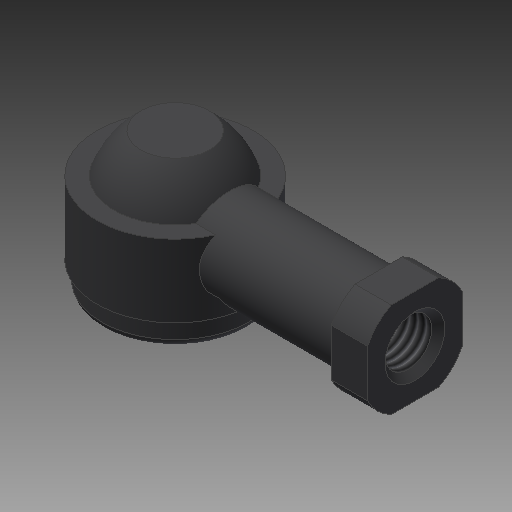
# Autodesk Inventor part: LHSA 10 Body1
Saved by Autodesk Inventor 2018 (Build 220112000, 112)
## iProperties
Category: PARTsolutions
Company: IKO
Created: 2017-10-01
Part Number: LHSA 10 Body1
Catalog Web Link: www.cadenas.de
Description: LHSA B1-
Vendor: IKO
Document SubType Name: Modeling
Designer: psAdmin
Manufacturer: IKO
Mass: 10.6246 g
Surface Area: 72.686 cm^2
Volume: 10.6246 cm^3
Density: 1 g/cm^3
Material: 一般
Appearance: PSOLRGB-128-128-128
PSOL_IDENT_0: {$CADENAS_DATA\23d-libs\iko\iko_bearings\l_balls\lhsa_body.prj},169 {VTYP=3D},{NB=LHSA 10 Body1},{LI
PSOL_IDENT_1: NA=LHSA 10 Body1},{NN=LHSA B1},{DATE=13.10.2016 10:02:12},{GEOMDATE=06.12.2007 08:55:00},{VERSION=},
PSOL_IDENT_2: {LINEID=60},{LINESUBID=-1},{WBVAR=}  {NB=LHSA 10 Body1},{LINA=LHSA 10 Body1},{KT=DUMMY},{IDNR=},{ORD
PSOL_IDENT_3: ER=LHSA 10},{VERS=3},{RID=G_50},{STDRT=10},{DESCR=LHSA},{TRNUMBER=},{PAST=A},{REST=O},{MASS=106},{S=
PSOL_IDENT_4: M10x1.25},{KDM=8.647},{NDM=10.000},{P1=1.250},{V=10},{D=28},{L=57.0},{L1=43},{L2=23},{SL1=6.5},{W=17
PSOL_IDENT_5: },{W1=17},{W2=17},{D1=15.0},{D2=19},{LL=49.0},{P=12.0},{LL1=16.0},{LL2=21.0},{LL3=17.0},{SDK=19.050}
PSOL_IDENT_6: ,{V1=11.0},{D3=12.2475},{D4=21.2001},{D5=26.3},{D6=25.65},{L3=53.8825},{L4=26.1906},{L5=28.5},{L12=3
PSOL_IDENT_7: 0.1645},{B=8.5},{B1=5.0},{B2=6.5},{B3=11.5},{B4=13.0},{B5=17.5073},{LL4=4.5},{LL5=9.0},{CB=0.0},{CC=
PSOL_IDENT_8: 0.9},{E=0},{F=0.0},{C1=1.1765},{C2=1.0},{R1=5},{R2=34.5114},{R3=15.7},{R4=1.3},{CS=7400},{SS1=8.160}
PSOL_IDENT_9: ,{S1=10},{LX=25},{LX1=28.0},{BL=3},{SC=1}
NN: LHSA B1
NB: LHSA 10 Body1
NBSYN: $ORDER. Body1
LINA: LHSA 10 Body1
ORDER: LHSA 10
VERS: 3
RID: G_50
STDRT: 10
DESCR: LHSA
PAST: A
REST: O
MASS: 106
S: M10x1.25
NDM: 10.000
P1: 1.250
V: 10
D: 28
L: 57.0
L1: 43
L2: 23
SL1: 6.5
W: 17
W1: 17
W2: 17
D1: 15.0
D2: 19
LL: 49.0
P: 12.0
LL1: 16.0
LL2: 21.0
LL3: 17.0
SDK: 19.050
V1: 11.0
D3: 12.2475
D4: 21.2001
D5: 26.3
D6: 25.65
L3: 53.8825
L4: 26.1906
L5: 28.5
L12: 30.1645
B: 8.5
B1: 5.0
B2: 6.5
B3: 11.5
B4: 13.0
B5: 17.5073
LL4: 4.5
LL5: 9.0
CB: 0.0
CC: 0.9
E: 0
F: 0.0
C1: 1.1765
C2: 1.0
R1: 5
R2: 34.5114
R3: 15.7
R4: 1.3
CS: 7400
SS1: 8.160
S1: 10
LX: 25
LX1: 28.0
BL: 3
SC: 1
SUPPLIER: IKO
ARTICLENO: LHSA 10 Body1
BOMINFO: LHSA 10 Body1
CREATOR: CADENAS GmbH
Title: LHSA 10 Body1
Author: Cadenas PARTsolutions
Autodesk Inventor part; units mm, degrees
sketch "Sketch_2" plane through (0, 0, 0) normal (0, 0, 1) x (1, 0, 0)
  line L0 (43, 16) -> (0, 16)
  line L1 (0, 16) -> (0, 23.5)
  line L2 (0, 23.5) -> (36.5, 23.5)
  line L3 (36.5, 23.5) -> (36.5, 25.5)
  line L4 (36.5, 25.5) -> (43, 25.5)
  line L5 (43, 25.5) -> (43, 16)
  line L6 (43, 16) -> (0, 16)
  constraints: 14 end point
revolve "Revolution1" add sketch "Sketch_2" angle 360 about axis through (43, 16, 0) along (1, 0, 0)
sketch "Sketch_16" plane through (0, 0, 0) normal (0, 0, 1) x (1, 0, 0)
  line L0 (-14, 12.5) -> (-14, 4.7)
  line L1 (-14, 4.7) -> (45.85, 4.7)
  line L2 (45.85, 4.7) -> (45.85, 27.3)
  line L3 (45.85, 27.3) -> (16.8094, 27.3)
  line L4 (16.8094, 27.3) -> (16.8094, 23.5)
  line L5 (16.8094, 23.5) -> (36.5, 23.5)
  line L6 (36.5, 23.5) -> (36.5, 24.5)
  line L7 (36.5, 24.5) -> (43, 24.5)
  line L8 (43, 24.5) -> (43, 7.5)
  line L9 (43, 7.5) -> (36.5, 7.5)
  line L10 (36.5, 7.5) -> (36.5, 8.5)
  line L11 (36.5, 8.5) -> (16.8094, 8.5)
  line L12 (16.8094, 8.5) -> (14.5, 12.5)
  line L13 (14.5, 12.5) -> (-14, 12.5)
  constraints: 28 end point
extrude "Extrusion1" cut sketch "Sketch_16" along normal mid plane 38
sketch "Sketch_12" plane through (0, 0, 0) normal (0, 0, 1) x (1, 0, 0)
  line L0 (0, 9.5) -> (0, 28)
  line L1 (0, 28) -> (6.1238, 28)
  arc A0 (10.8825, 21) -> (6.1238, 28) centre (-4.0001, 16.0001) ccw
  line L2 (10.8825, 21) -> (14, 21)
  line L3 (14, 21) -> (14, 12.5)
  line L4 (14, 12.5) -> (12.825, 12.5)
  line L5 (12.825, 12.5) -> (12.825, 9.5)
  line L6 (12.825, 9.5) -> (0, 9.5)
  line L7 (0, 9.5) -> (0, 28)
  constraints: 16 end point, 2 point on circle, 1 centre point
revolve "Revolution2" add sketch "Sketch_12" angle 360 about axis through (0, 9.5, 0) along (0, -1, 0)
sketch "Sketch_13" plane through (0, 0, 0) normal (0, 0, 1) x (1, 0, 0)
  line L0 (9.525, 16) -> (-9.525, 16)
  arc A0 (9.525, 16) -> (-9.525, 16) centre (0, 16) ccw
  line L1 (9.525, 16) -> (-9.525, 16)
  constraints: 4 end point, 2 point on circle, 1 centre point
revolve "Revolution3" cut sketch "Sketch_13" angle 360 about axis through (9.525, 16, 0) along (1, 0, 0)
sketch "Sketch_14" plane through (0, 0, 0) normal (0, 0, 1) x (1, 0, 0)
  line L0 (0, 9.5) -> (0, 14.5)
  line L1 (0, 14.5) -> (10.6001, 14.5)
  line L2 (10.6001, 14.5) -> (10.6001, 9.5)
  line L3 (10.6001, 9.5) -> (0, 9.5)
  line L4 (0, 9.5) -> (0, 14.5)
  constraints: 10 end point
revolve "Revolution4" cut sketch "Sketch_14" angle 360 about axis through (0, 9.5, 0) along (0, -1, 0)
sketch "Sketch_15" plane through (0, 0, 0) normal (0, 0, 1) x (1, 0, 0)
  line L0 (0, 9.5) -> (0, 14.5)
  line L1 (6.9624, 9.5) -> (10.6001, 9.5)
  line L2 (10.6001, 9.5) -> (10.6001, 14.5)
  line L3 (10.6001, 14.5) -> (9.4061, 14.5)
  arc A0 (6.9624, 9.5) -> (9.4061, 14.5) centre (0, 16) ccw
  constraints: 8 end point, 2 point on circle, 1 centre point
revolve "Revolution5" add sketch "Sketch_15" angle 360 about axis through (0, 9.5, 0) along (0, -1, 0)
sketch "Sketch_17" plane through (0, 0, 0) normal (0, 0, 1) x (1, 0, 0)
  line L0 (0, 4.5) -> (0, 12.5)
  line L1 (5.5, 5.4) -> (5.5, 4.5)
  line L2 (5.5, 4.5) -> (6, 4.5)
  line L3 (6, 4.5) -> (11.85, 3.4927)
  arc A0 (11.85, 3.4927) -> (13.15, 4.7927) centre (11.85, 4.7927) ccw
  line L4 (13.15, 4.7927) -> (13.15, 8)
  line L5 (13.15, 8) -> (14, 8)
  line L6 (14, 8) -> (14, 12.5)
  line L7 (14, 12.5) -> (12.825, 12.5)
  line L8 (12.825, 12.5) -> (12.825, 9.5)
  line L9 (12.825, 9.5) -> (12.25, 9.5)
  line L10 (12.25, 9.5) -> (12.25, 5.6927)
  arc A1 (10.95, 4.3927) -> (12.25, 5.6927) centre (10.95, 5.6927) ccw
  line L11 (10.95, 4.3927) -> (6, 5.4)
  line L12 (6, 5.4) -> (5.5, 5.4)
  constraints: 26 end point, 4 point on circle, 2 centre point
revolve "Revolution6" add sketch "Sketch_17" angle 360 about axis through (0, 4.5, 0) along (0, -1, 0)
sketch "Sketch8" plane through (43, 16, 0) normal (1, 0, 0) x (0, 0, -1)
  point P0 (0, 0)
hole "Hole1" at (43, 16, 0) direction (-1, 0, 0) diameter 8.376 depth 26.1765 tip angle 120 countersink diameter 10.729 countersink angle 90 thread size "M10x1.5" class "6H" standard "ISO Metric profile"
sketch "Sketch_20" plane through (36.5, 0, 0) normal (1, 0, 0) x (0, 0, -1)
  line L0 (-12.75, 5.8) -> (12.75, 5.8)
  line L1 (12.75, 5.8) -> (12.75, 26.2)
  line L2 (12.75, 26.2) -> (-12.75, 26.2)
  line L3 (-12.75, 26.2) -> (-12.75, 5.8)
  line L4 (-8.5, 24.5) -> (-8.5, 7.5)
  line L5 (-8.5, 7.5) -> (8.5, 7.5)
  line L6 (8.5, 7.5) -> (8.5, 24.5)
  line L7 (8.5, 24.5) -> (-8.5, 24.5)
  constraints: 16 end point
extrude "Extrusion2" cut sketch "Sketch_20" along normal blind 6.5
ref_plane "IP1_XY" through (0, 16, 0) normal (0, 0, 1) x (1, 0, 0)
ref_plane "IP1_YZ" through (0, 16, 0) normal (1, 0, 0) x (0, 1, 0)
ref_plane "IP1_ZX" through (0, 16, 0) normal (0, 1, 0) x (0, 0, 1)
body "Solid1"
